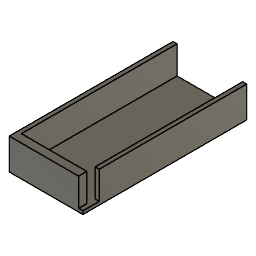
supporto_batteria_parametrico (Autodesk Fusion 360 design; units mm, degrees)
part number: 2026-07-13-18-12-15-809
part number: 2026-07-13-18-12-16-008
Autodesk Fusion 360 part; units mm, degrees
sketch "Schizzo1" plane through (0, 0, 0) normal (0, 0, 1) x (1, 0, 0) in component "01_Supporto_batteria_parametrico"
  line L0 (-22.5, -50) -> (22.5, -50)
  line L1 (22.5, -50) -> (22.5, 50)
  line L2 (22.5, 50) -> (-22.5, 50)
  line L3 (-22.5, 50) -> (-22.5, -50)
extrude "Estrusione_Fondo_supporto_batteria" add sketch "Schizzo1" along normal blind 2 in component "01_Supporto_batteria_parametrico"
ref_plane "Piano di lavoro1" through (0, 0, 2) normal (0, 0, 1) x (1, 0, 0) in component "01_Supporto_batteria_parametrico"
sketch "Schizzo2" plane through (0, 0, 2) normal (0, 0, 1) x (1, 0, 0) in component "01_Supporto_batteria_parametrico"
  line L0 (-22.5, -50) -> (-20, -50)
  line L1 (-20, -50) -> (-20, 50)
  line L2 (-20, 50) -> (-22.5, 50)
  line L3 (-22.5, 50) -> (-22.5, -50)
extrude "Estrusione_Parete_lunga_Ovest" add sketch "Schizzo2" along normal blind 17 in component "01_Supporto_batteria_parametrico"
sketch "Schizzo3" plane through (0, 0, 2) normal (0, 0, 1) x (1, 0, 0) in component "01_Supporto_batteria_parametrico"
  line L0 (20, -50) -> (22.5, -50)
  line L1 (22.5, -50) -> (22.5, 50)
  line L2 (22.5, 50) -> (20, 50)
  line L3 (20, 50) -> (20, -50)
extrude "Estrusione_Parete_lunga_Est" add sketch "Schizzo3" along normal blind 17 in component "01_Supporto_batteria_parametrico"
sketch "Schizzo4" plane through (0, 0, 2) normal (0, 0, 1) x (1, 0, 0) in component "01_Supporto_batteria_parametrico"
  line L0 (-22.5, -50) -> (22.5, -50)
  line L1 (22.5, -50) -> (22.5, -45)
  line L2 (22.5, -45) -> (-22.5, -45)
  line L3 (-22.5, -45) -> (-22.5, -50)
extrude "Estrusione_Parete_corta_chiusa" add sketch "Schizzo4" along normal blind 17 in component "01_Supporto_batteria_parametrico"
sketch "Schizzo5" plane through (0, 0, 2) normal (0, 0, 1) x (1, 0, 0) in component "01_Supporto_batteria_parametrico"
  line L0 (19.9, -50) -> (22.6, -50)
  line L1 (22.6, -50) -> (22.6, -40)
  line L2 (22.6, -40) -> (19.9, -40)
  line L3 (19.9, -40) -> (19.9, -50)
extrude "Apertura_cavi_parete_lunga_Est" cut sketch "Schizzo5" along normal blind 17 in component "01_Supporto_batteria_parametrico"
component "01_Supporto_batteria_parametrico" placed x (1, 0, 0) y (0, 1, 0) z (0, 0, 1) at (0, 0, 0)
equation "batt_vano_lunghezza = 95.0 mm" comment "Vano batteria"
equation "batt_vano_larghezza = 40.0 mm" comment "Vano batteria"
equation "batt_esterno_lunghezza = 100.0 mm" comment "Supporto batteria"
equation "batt_esterno_larghezza = 45.0 mm" comment "Supporto batteria"
equation "batt_fondo_spessore = 2.0 mm" comment "Fondo supporto batteria"
equation "batt_parete_spessore = 2.5 mm" comment "Pareti laterali"
equation "batt_parete_altezza = 17.0 mm" comment "Pareti laterali"
equation "batt_apertura_cavi = 10.0 mm" comment "Passaggio cavi"
equation "d9 = batt_fondo_spessore"
equation "d11 = batt_fondo_spessore"
equation "d13 = batt_parete_altezza"
equation "d15 = batt_parete_altezza"
equation "d17 = batt_parete_altezza"
equation "d19 = batt_parete_altezza"
named bodies: "Supporto_batteria_con_apertura_cavi"
